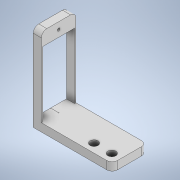
# Autodesk Inventor part: Part3
Saved by Autodesk Inventor 2022 (Build 260153000, 153)
## iProperties
Created: 2021-10-11
Part Number: Part3
Material: Generic
Document SubType Name: Modeling
Designer: Route
Density: 1 g/cm^3
Appearance: Default
Author: Route
Autodesk Inventor part; units mm, degrees
ref_plane "YZ Plane" through (0, 0, 0) normal (1, 0, 0) x (0, 1, 0)
ref_plane "XZ Plane" through (0, 0, 0) normal (0, 1, 0) x (-1, 0, 0)
ref_plane "XY Plane" through (0, 0, 0) normal (0, 0, 1) x (1, 0, 0)
sketch "Sketch1" plane through (0, 0, 0) normal (0, 1, 0) x (-1, 0, 0)
  line L0 (29.21, 0) -> (29.21, 12.8)
  line L1 (29.21, 12.8) -> (0, 12.8)
  line L2 (29.21, 12.8) -> (13.21, 12.8)
  circle A0 centre (3.3025, 9.6) radius 1.5
  circle A1 centre (9.9075, 9.6) radius 1.5
  line L3 (0, 12.8) -> (0, 0)
  line L4 (0, 0) -> (29.21, 0)
  dimension "d0" = 12.8
  dimension "d1" = 16
  dimension "d4" = 3
  dimension "d5" = 3
  constraints: 10 end point, 2 centre point, 2 perpendicular, 1 point on line, 1 vertical
  measures "d0" distance of L0.start L2.start
  measures "d1" distance of L2.start L2.end
  measures "d4" diameter of A0
  measures "d5" diameter of A1
extrude "Extrusion1" add sketch "Sketch1" along normal blind 3
sketch "Sketch2" plane through (0, 3, 0) normal (0, 1, 0) x (1, 0, 0)
  line L0 (0, 0) -> (-29.21, 0) projected
  line L1 (-29.21, -12.8) -> (0, -12.8) projected
  line L2 (-29.21, 0) -> (-26.21, 0)
  line L3 (-26.21, 0) -> (-26.21, -12.8)
  line L4 (-26.21, -12.8) -> (-29.21, -12.8)
  line L5 (-29.21, -12.8) -> (-29.21, 0)
  dimension "d8" = 3
  constraints: 8 end point, 2 parallel, 1 horizontal, 1 perpendicular, 1 point on line
  measures "d8" distance of L3.end L4.end
extrude "Extrusion2" add sketch "Sketch2" along normal blind 29.2
sketch "Sketch3" plane through (-29.21, 0, 0) normal (-1, 0, 0) x (0, 0, 1)
  line L0 (12.8, 0) -> (12.8, 32.2) projected
  line L1 (12.8, 16.1) -> (0, 16.1)
  line L2 (0, 0) -> (0, 32.2) projected
  line L3 (6.4, 27.2) -> (12.3, 27.2)
  line L4 (12.3, 27.2) -> (12.3, 5)
  line L5 (12.3, 5) -> (0.5, 5)
  line L6 (0.5, 5) -> (0.5, 27.2)
  line L7 (0.5, 27.2) -> (6.4, 27.2)
  line L8 (0, 0) -> (12.8, 0) projected
  circle A0 centre (6.4, 2.5) radius 0.5
  line L9 (0, 32.2) -> (12.8, 32.2) projected
  circle A1 centre (6.4, 29.7) radius 0.5
  dimension "d12" = 5.9
  dimension "d13" = 11.8
  dimension "d14" = 1
  dimension "d15" = 1
  constraints: 12 end point, 4 perpendicular, 2 centre point, 2 midpoint, 1 point on line
  measures "d12" distance of L3.start L3.end
  measures "d13" distance of L4.end L5.end
  measures "d14" diameter of A0
  measures "d15" diameter of A1
extrude "Extrusion3" cut sketch "Sketch3" against normal blind 3 contours L4 L5 L6 L1 | L1 L6 L7 L3 L4 | A0 | A1
fillet "Fillet1" radius 2 2 edges at (-27.71, 32.2, 12.8) (-27.71, 32.2, 0)
fillet "Fillet2" radius 2 2 edges at (0, 1.5, 0) (0, 1.5, 12.8)
sketch "Эскиз4" plane through (-26.21, 3, 12.8) normal (1, 0, 0) x (0, 0, -1)
  line L0 (12.3, 2) -> (0.5, 2) projected
  line L1 (12.3, 2) -> (0.5, 2)
  line L2 (0.5, 2) -> (0.5, 0)
  line L3 (0, 0) -> (2, 0) projected
  line L4 (12.3, 2) -> (12.3, 0)
  line L5 (12.8, 0) -> (6.4, 0) projected
  line L6 (12.3, 0) -> (0.5, 0)
  point P0 (12.8, -3)
  constraints: 8 end point, 2 perpendicular, 2 point on line, 1 horizontal, 1 parallel
extrude "Выдавливание4" cut sketch "Эскиз4" against normal blind 32.2
body "Solid1"
